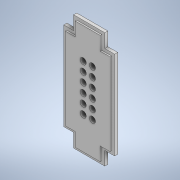
# Autodesk Inventor part: rib
Saved by Autodesk Inventor 2021 (Build 250183000, 183)
## iProperties
Created: 2020-11-25
Part Number: rib
Material: Generic
Document SubType Name: Modeling
Designer: Admin
Density: 1 g/cm^3
Appearance: Default
Mass: 47.3201 g
Surface Area: 212.307 cm^2
Volume: 47.3201 cm^3
Author: Admin
Autodesk Inventor part; units mm, degrees
ref_plane "YZ Plane" through (0, 0, 0) normal (1, 0, 0) x (0, 1, 0)
ref_plane "XZ Plane" through (0, 0, 0) normal (0, 1, 0) x (-1, 0, 0)
ref_plane "XY Plane" through (0, 0, 0) normal (0, 0, 1) x (1, 0, 0)
sketch "Sketch1" plane through (0, 0, 0) normal (0, 0, 1) x (1, 0, 0)
  line L0 (-39.7468, 54.4174) -> (-39.7468, -52.4226)
  line L1 (-39.7468, -52.4226) -> (-26.9468, -52.4226)
  line L2 (-26.9468, -52.4226) -> (-26.9468, -70.2026)
  line L3 (-26.9468, -70.2026) -> (5.6532, -70.2026)
  line L4 (5.6532, -70.2026) -> (5.6532, -52.4226)
  line L5 (5.6532, -52.4226) -> (18.4532, -52.4226)
  line L6 (18.4532, -52.4226) -> (18.4532, 54.4174)
  line L7 (18.4532, 54.4174) -> (5.6532, 54.4174)
  line L8 (5.6532, 54.4174) -> (5.6532, 72.1974)
  line L9 (5.6532, 72.1974) -> (-26.9468, 72.1974)
  line L10 (-26.9468, 72.1974) -> (-26.9468, 54.4174)
  line L11 (-39.7468, 54.4174) -> (-26.9468, 54.4174)
  line L12 (-23.8279, 76.1974) -> (9.6532, 76.1974)
  line L13 (9.6532, 76.1974) -> (9.6532, 58.4174)
  line L14 (9.6532, 58.4174) -> (22.4532, 58.4174)
  line L15 (22.4532, 58.4174) -> (22.4532, -56.4226)
  line L16 (22.4532, -56.4226) -> (9.6532, -56.4226)
  line L17 (9.6532, -56.4226) -> (9.6532, -74.2026)
  line L18 (9.6532, -74.2026) -> (-30.9468, -74.2026)
  line L19 (-30.9468, -74.2026) -> (-30.9468, -56.4226)
  line L20 (-30.9468, -56.4226) -> (-43.7468, -56.4226)
  line L21 (-43.7468, -56.4226) -> (-43.7468, 58.4174)
  line L22 (-43.7468, 58.4174) -> (-30.9468, 58.4174)
  line L23 (-30.9468, 76.1974) -> (-23.8279, 76.1974)
  line L24 (-30.9468, 58.4174) -> (-30.9468, 76.1974)
  point P0 (0, 0)
  dimension "d0" = 106.84
  dimension "d1" = 142.4
  dimension "d2" = 17.78
  dimension "d3" = 17.78
  dimension "d4" = 32.6
  dimension "d5" = 12.8
  dimension "d6" = 12.8
  dimension "d7" = 4
  dimension "d8" = 4
  dimension "d9" = 4
  dimension "d10" = 4
  dimension "d11" = 4
  dimension "d12" = 4
  dimension "d13" = 4
  dimension "d14" = 4
  dimension "d15" = 4
  constraints: 50 end point, 16 perpendicular, 16 point on line, 1 horizontal, 1 parallel, 1 vertical
  measures "d0" distance of L0.start L0.end
  measures "d1" distance between parallel lines of L3 L9
  measures "d2" distance of L9.end L10.end
  measures "d3" distance of L1.end L2.end
  measures "d4" distance of L8.end L9.end
  measures "d5" distance of L0.start L10.end
  measures "d6" distance of L6.end L7.end
  measures "d7" distance between parallel lines of L9 L12
  measures "d8" distance between parallel lines of L13 L8
  measures "d9" distance between parallel lines of L10 L24
  measures "d10" distance between parallel lines of L11 L22
  measures "d11" distance between parallel lines of L7 L14
  measures "d12" distance between parallel lines of L0 L21
  measures "d13" distance between parallel lines of L6 L15
  measures "d14" distance between parallel lines of L1 L20
  measures "d15" distance between parallel lines of L18 L3
sketch "Sketch2" plane through (0, 0, 0) normal (0, 0, 1) x (1, 0, 0)
  circle A0 centre (-4.4728, 32.0701) radius 4
  circle A1 centre (-16.4728, 32.0701) radius 4
  circle A2 centre (-4.4728, 20.0701) radius 4
  circle A3 centre (-16.4728, 20.0701) radius 4
  circle A4 centre (-4.4728, 8.0701) radius 4
  circle A5 centre (-16.4728, 8.0701) radius 4
  circle A6 centre (-4.4728, -3.9299) radius 4
  circle A7 centre (-16.4728, -15.9299) radius 4
  circle A8 centre (-4.4728, -15.9299) radius 4
  circle A9 centre (-16.4728, -3.9299) radius 4
  circle A10 centre (-4.4728, -27.9299) radius 4
  circle A11 centre (-16.4728, -27.9299) radius 4
  point P0 (0, 0)
  dimension "d22" = 8
  dimension "d27" = 8
  dimension "d30" = 8
  dimension "d34" = 8
  dimension "d38" = 8
  dimension "d42" = 8
  dimension "d59" = 12
  dimension "d63" = 12
  dimension "d67" = 12
  dimension "d70" = 12
  dimension "d71" = 12
  dimension "d75" = 12
  dimension "d93" = 12
  dimension "d94" = 0
  dimension "d97" = 0
  dimension "d98" = 12
  dimension "d102" = 0
  dimension "d103" = 12
  constraints: 12 centre point
  measures "d22" diameter of A1
  measures "d27" diameter of A3
  measures "d30" diameter of A5
  measures "d34" diameter of A7
  measures "d38" diameter of A9
  measures "d42" diameter of A11
  measures "d59" distance of A1.centre A0.centre
  measures "d63" distance of A3.centre A1.centre
  measures "d67" distance of A3.centre A2.centre
  measures "d70" distance of A5.centre A3.centre
  measures "d71" distance of A4.centre A2.centre
  measures "d75" distance of A5.centre A4.centre
  measures "d93" distance of A6.centre A9.centre
  measures "d94" vertical distance of A9.centre A6.centre
  measures "d97" vertical distance of A7.centre A8.centre
  measures "d98" distance of A7.centre A8.centre
  measures "d102" vertical distance of A11.centre A10.centre
  measures "d103" distance of A11.centre A10.centre
extrude "Extrusion1" add sketch "Sketch1" along normal blind 6 contours L11 L10 L9 L8 L7 L6 L5 L4 L3 L2 L1 L0
extrude "Extrusion2" add sketch "Sketch1" along normal blind 4
extrude "Extrusion3" cut sketch "Sketch2" along normal blind 12
body "Solid1"
